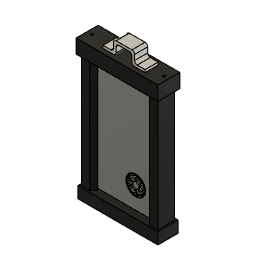
Beskar ingot holder v2 (Autodesk Fusion 360 design; units mm, degrees)
Autodesk Fusion 360 part; units mm, degrees
sketch "Sketch1" plane through (0, 0, 0) normal (0, 1, 0) x (1, 0, 0)
  line L0 (37.5, 3.5) -> (-37.5, 3.5)
  line L1 (-37.5, 3.5) -> (-37.5, -3.5)
  line L2 (-37.5, -3.5) -> (37.5, -3.5)
  line L3 (37.5, -3.5) -> (37.5, 3.5)
  line L4 (37.5, 3.5) -> (-37.5, -3.5) construction
  line L5 (-37.5, 3.5) -> (37.5, -3.5) construction
  line L6 (-43.5, -9.5) -> (43.5, -9.5)
  line L7 (43.5, -9.5) -> (43.5, 9.5)
  line L8 (43.5, 9.5) -> (-43.5, 9.5)
  line L9 (-43.5, 9.5) -> (-43.5, -9.5)
  line L10 (-43.5, 9.5) -> (-36.2124, 9.5)
  line L11 (-36.2124, 9.5) -> (-36.2124, 7.7353)
  line L12 (-36.2124, 7.7353) -> (-43.5, 7.7353)
  line L13 (-43.5, 7.7353) -> (-43.5, 9.5)
  line L14 (-43.5, 9.5) -> (-36.2124, 7.7353) construction
  line L15 (-36.2124, 9.5) -> (-43.5, 7.7353) construction
  line L16 (47, -6) -> (40, -6)
  line L17 (40, -6) -> (40, -13)
  line L18 (40, -13) -> (47, -13)
  line L19 (47, -13) -> (47, -6)
  line L20 (47, -6) -> (40, -13) construction
  line L21 (40, -6) -> (47, -13) construction
  line L22 (47, 6) -> (40, 6)
  line L23 (40, 6) -> (40, 13)
  line L24 (40, 13) -> (47, 13)
  line L25 (47, 13) -> (47, 6)
  line L26 (47, 6) -> (40, 13) construction
  line L27 (40, 6) -> (47, 13) construction
  line L28 (-40, -13) -> (-47, -13)
  line L29 (-47, -13) -> (-47, -6)
  line L30 (-47, -6) -> (-40, -6)
  line L31 (-40, -6) -> (-40, -13)
  line L32 (-40, -13) -> (-47, -6) construction
  line L33 (-47, -13) -> (-40, -6) construction
  line L34 (-40, 6) -> (-47, 6)
  line L35 (-47, 6) -> (-47, 13)
  line L36 (-47, 13) -> (-40, 13)
  line L37 (-40, 13) -> (-40, 6)
  line L38 (-40, 6) -> (-47, 13) construction
  line L39 (-47, 6) -> (-40, 13) construction
  line L40 (0, 0) -> (-0.7931, -0.074)
  circle A0 centre (0, 0) radius 15
  circle A1 centre (15, 0) radius 1.99
  circle A2 centre (-15, 0) radius 1.99
  line L41 (-37.5, 0) -> (-41, 0)
  line L42 (37.5, 0) -> (41, 0)
  circle A3 centre (41, 0) radius 1.5
  circle A4 centre (-41, 0) radius 1.5
  line L43 (-46.5, -12.5) -> (46.5, -12.5)
  line L44 (46.5, -12.5) -> (46.5, 12.5)
  line L45 (46.5, 12.5) -> (-46.5, 12.5)
  line L46 (-46.5, 12.5) -> (-46.5, -12.5)
  point P0 (-39.8562, 8.6177)
  point P1 (43.5, -9.5)
  point P2 (43.5, 9.5)
  point P3 (-43.5, -9.5)
  point P4 (-43.5, 9.5)
  dimension "d1" = 75
  dimension "d2" = 7
  dimension "d3" = 6
  dimension "d4" = 7
  dimension "d5" = 7
  dimension "d6" = 7
  dimension "d7" = 7
  dimension "d8" = 7
  dimension "d9" = 7
  dimension "d10" = 7
  dimension "d11" = 7
  dimension "d26" = 30
  dimension "d27" = 3.98
  dimension "d28" = 3.98
  dimension "d31" = 3.5
  dimension "d32" = 3.5
  dimension "d33" = 3
  dimension "d34" = 3
  dimension "d66" = 9
  constraint horizontal L0
  constraint perpendicular L0 L1
  constraint parallel L0 L2
  constraint parallel L1 L3
  constraint coincident L4 L40.start
  constraint coincident L5 L40.start
  constraint coincident L40.start A0.centre
  constraint horizontal L10
  constraint perpendicular L10 L11
  constraint parallel L10 L12
  constraint parallel L11 L13
  constraint coincident L14 P0
  constraint coincident L15 P0
  constraint horizontal L16
  constraint perpendicular L16 L17
  constraint parallel L16 L18
  constraint parallel L17 L19
  constraint coincident L20 P1
  constraint coincident L21 P1
  constraint coincident P1 L6.end
  constraint horizontal L22
  constraint perpendicular L22 L23
  constraint parallel L22 L24
  constraint parallel L23 L25
  constraint coincident L26 P2
  constraint coincident L27 P2
  constraint coincident P2 L7.end
  constraint horizontal L28
  constraint perpendicular L28 L29
  constraint parallel L28 L30
  constraint parallel L29 L31
  constraint coincident L32 P3
  constraint coincident L33 P3
  constraint coincident P3 L6.start
  constraint horizontal L34
  constraint perpendicular L34 L35
  constraint parallel L34 L36
  constraint parallel L35 L37
  constraint coincident L38 P4
  constraint coincident L39 P4
  constraint coincident P4 L8.end
  constraint coincident L4 L40.end
  constraint coincident A0 A1.centre
  constraint coincident A0 A2.centre
  constraint midpoint L1 L41.start
  constraint perpendicular L1 L41
  constraint midpoint L3 L42.start
  constraint perpendicular L7 L42
  constraint coincident L42.end A3.centre
  constraint coincident L41.end A4.centre
  measures "d1" distance of L1.end L2.end
  measures "d2" distance of L0.end L1.end
  measures "d4" distance of L17.end L18.end
  measures "d5" distance of L16.end L17.end
  measures "d6" distance of L23.end L24.end
  measures "d7" distance of L22.end L23.end
  measures "d8" distance of L29.end L30.end
  measures "d9" distance of L28.end L29.end
  measures "d10" distance of L35.end L36.end
  measures "d11" distance of L34.end L35.end
  measures "d26" diameter of A0
  measures "d27" diameter of A1
  measures "d28" diameter of A2
  measures "d31" distance of L41.start L41.end
  measures "d32" distance of L42.start L42.end
  measures "d33" diameter of A3
  measures "d34" diameter of A4
extrude "Extrude1" add sketch "Sketch1" along normal blind 7 contours L0 L2 L3 L6 L7 L8 L16 L17 L22 L23 A0 | L0 L8 A0 | L0 L1 L2 L6 L8 L9 L11 L12 L30 L31 L34 L37 A0 | L7 L8 L22 L23 | L2 L6 A0 | L8 L10 L11 L12 L37 | L8 L9 L10 L12 L13 L37 | L6 L7 L16 L17 | L9 L12 L34 L37 | L6 L9 L30 L31 | A3 | A4 makes body 1
extrude "Extrude2" add sketch "Sketch1" 1 faces at (-3.8694, 0, 5.5) against normal blind 6 contours L0 L2 L3 A0 A1 | L0 L2 L3 L6 L7 L8 L16 L17 L22 L23 A0 | L0 L2 A0 A1 A2 | L0 L8 A0 | L0 L1 L2 A0 A2 | L0 L1 L2 L6 L8 L9 L11 L12 L30 L31 L34 L37 A0 | A0 A1 | A0 A1 | A0 A2 | A0 A2 | L7 L8 L22 L23 | L2 L6 A0 | L8 L10 L11 L12 L37 | L8 L9 L10 L12 L13 L37 | L6 L7 L16 L17 | L9 L12 L34 L37 | L6 L9 L30 L31 | A3 | A4 on bodies 1 bodies 1
sketch "Sketch2" plane through (0, 7, 0) normal (0, 1, 0) x (-1, 0, 0)
  line L0 (-37.5, -3.5) -> (-37.5, 3.5)
  line L1 (-37.5, 3.5) -> (37.5, 3.5)
  line L2 (37.5, 3.5) -> (37.5, -3.5)
  line L3 (37.5, -3.5) -> (-37.5, -3.5)
  line L4 (43.5, -9.5) -> (43.5, 9.5)
  line L5 (43.5, 9.5) -> (-43.5, 9.5)
  line L6 (-43.5, 9.5) -> (-43.5, -9.5)
  line L7 (-43.5, -9.5) -> (43.5, -9.5)
  line L8 (-43.5, -3.5) -> (43.5, -3.5)
  line L9 (-43.5, 3.5) -> (43.5, 3.5)
  line L10 (-43.5, -5) -> (43.5, -5)
  line L11 (-43.5, 4.9996) -> (43.5, 4.9996)
  line L12 (-37.5, 4.9996) -> (-37.5, -5)
  line L13 (37.5, 4.9996) -> (37.5, -5)
  line L14 (43.5, -9.5) -> (29.5, -9.5)
  line L15 (29.5, -9.5) -> (29.5, 9.5)
  line L16 (29.5, 9.5) -> (43.5, 9.5)
  line L17 (43.5, 9.5) -> (43.5, -9.5)
  line L18 (-43.5, 9.5) -> (-29.5, 9.5)
  line L19 (-29.5, 9.5) -> (-29.5, -9.5)
  line L20 (-29.5, -9.5) -> (-43.5, -9.5)
  line L21 (-43.5, -9.5) -> (-43.5, 9.5)
  dimension "d16" = 1.5
  dimension "d17" = -1.4996
  dimension "d46" = 14
  dimension "d47" = 14
  constraint coincident L6 L8.start
  constraint coincident L4 L8.end
  constraint perpendicular L4 L8
  constraint coincident L6 L9.start
  constraint coincident L4 L9.end
  constraint perpendicular L4 L9
  constraint coincident L11 L12.start
  constraint coincident L10 L12.end
  constraint perpendicular L10 L12
  constraint coincident L11 L13.start
  constraint coincident L10 L13.end
  constraint perpendicular L10 L13
  constraint horizontal L14
  constraint vertical L15
  constraint horizontal L16
  constraint vertical L17
  constraint coincident L4.start L7.end
  constraint horizontal L18
  constraint vertical L19
  constraint horizontal L20
  constraint vertical L21
  constraint coincident L5.end L6.start
  measures "d46" distance of L4.start L14.end
  measures "d47" distance of L5.end L18.end
extrude "Extrude3" add sketch "Sketch2" along normal blind 132.5 separate body contours L0 L6 L8 L9 L12 L21 | L6 L8 L10 L12 L21 | L6 L9 L11 L12 L21 | L6 L7 L10 L19 L20 L21 | L5 L6 L11 L18 L19 L21 | L2 L4 L8 L9 L13 L17 | L4 L8 L10 L13 L17 | L4 L7 L10 L14 L15 L17 | L4 L9 L11 L13 L17 | L4 L5 L11 L15 L16 L17 makes body 2 at (-43.5, 51.1667, -3.1667) makes body 3 at (43.5, 51.1667, 3.1667)
extrude "Extrude4" add sketch "Sketch1" along normal blind 139 separate body contours L0 L2 L3 A0 A1 | L0 L2 A0 A1 A2 | L0 L1 L2 A0 A2 | A0 A1 | A0 A1 | A0 A2 | A0 A2 makes body 4
sketch "Sketch3" plane through (-43.5, 0, 0) normal (-1, 0, 0) x (0, 0, 1)
  line L0 (-9.5, -6) -> (9.5, -6)
  line L1 (-9.5, 142) -> (-4.5002, 142)
  line L2 (-4.5002, 142) -> (-4.5002, 137)
  line L3 (-4.5002, 137) -> (-9.5, 137)
  line L4 (-9.5, 137) -> (-9.5, 142)
  circle A0 centre (-4.5002, 137) radius 1.25
  line L5 (9.5, -6) -> (9.5, 7)
  line L6 (-9.5, 7) -> (-9.5, -6)
  line L7 (9.5, 7) -> (-9.5, 7)
  dimension "d22" = 5
  dimension "d23" = 2.5
  constraint horizontal L1
  constraint vertical L2
  constraint horizontal L3
  constraint vertical L4
  constraint coincident L2.end L3.start
  measures "d22" distance of L1.start L3.end
  measures "d23" diameter of A0
extrude "Extrude5" [suppressed]
extrude "Extrude6" cut sketch "Sketch1" along normal blind 10 and the other way blind 6 contours A3 | A4 bodies 1 3 2
extrude "Extrude7" add sketch "Sketch3" against normal blind 87 separate body contours L2 L3 A0 | L2 L3 A0 makes body 5
sketch "Sketch4" plane through (0, 0, -3.5) normal (0, 0, -1) x (-1, 0, 0)
  line L0 (-37.5, 0) -> (37.5, 0)
  line L1 (37.5, 0) -> (37.5, 139)
  line L2 (37.5, 139) -> (-37.5, 139)
  line L3 (-37.5, 139) -> (-37.5, 0)
  line L4 (-37.5, 139) -> (-12.5, 139)
  line L5 (-12.5, 139) -> (-12.5, 114)
  line L6 (-12.5, 114) -> (-37.5, 114)
  line L7 (-37.5, 114) -> (-37.5, 139)
  spline S0 degree 3 poles (-12.2923, 125.7038) (-6.1064, 125.7038) (-1.086, 120.6834) (-1.086, 114.4975) knots 0 0 0 0 1 1 1 1
  spline S1 degree 3 poles (-1.086, 114.4975) (-1.086, 108.3117) (-6.1064, 103.2912) (-12.2923, 103.2913) knots 0 0 0 0 1 1 1 1
  spline S2 degree 3 poles (-12.2923, 103.2913) (-18.4782, 103.2913) (-23.4986, 108.3117) (-23.4986, 114.4975) knots 0 0 0 0 1 1 1 1
  spline S3 degree 3 poles (-23.4986, 114.4975) (-23.4986, 120.6834) (-18.4782, 125.7038) (-12.2923, 125.7038) knots 0 0 0 0 1 1 1 1
  spline S4 degree 3 poles (-11.7634, 124.7747) (-11.7697, 124.7751) (-11.7762, 124.7744) (-11.7825, 124.7747) knots 0 0 0 0 1 1 1 1
  line L8 (-11.7825, 124.7747) -> (-11.8301, 124.0148)
  spline S5 degree 3 poles (-11.8301, 124.0148) (-11.1838, 123.984) (-10.5547, 123.8897) (-9.9481, 123.7361) knots 0 0 0 0 1 1 1 1
  line L9 (-9.9481, 123.7361) -> (-10.1363, 122.9952)
  spline S6 degree 3 poles (-10.1363, 122.9952) (-8.5442, 122.5919) (-7.1261, 121.7535) (-6.0149, 120.6129) knots 0 0 0 0 1 1 1 1
  line L10 (-6.0149, 120.6129) -> (-5.4694, 121.1465)
  spline S7 degree 3 poles (-5.4694, 121.1465) (-5.0257, 120.6913) (-4.629, 120.1913) (-4.283, 119.6552) knots 0 0 0 0 1 1 1 1
  line L11 (-4.283, 119.6552) -> (-3.6446, 120.0769)
  spline S8 degree 3 poles (-3.6446, 120.0769) (-5.3883, 122.773) (-8.3585, 124.602) (-11.7634, 124.7747) knots 0 0 0 0 1 1 1 1
  spline S9 degree 3 poles (-12.8021, 124.7747) (-16.2149, 124.6078) (-19.193, 122.778) (-20.94, 120.0769) knots 0 0 0 0 1 1 1 1
  line L12 (-20.94, 120.0769) -> (-20.3015, 119.6552)
  spline S10 degree 3 poles (-20.3015, 119.6552) (-19.9563, 120.19) (-19.56, 120.6899) (-19.1175, 121.1441) knots 0 0 0 0 1 1 1 1
  line L13 (-19.1175, 121.1441) -> (-18.572, 120.6129)
  spline S11 degree 3 poles (-18.572, 120.6129) (-17.4607, 121.7541) (-16.0409, 122.5918) (-14.4483, 122.9952) knots 0 0 0 0 1 1 1 1
  line L14 (-14.4483, 122.9952) -> (-14.6365, 123.7361)
  spline S12 degree 3 poles (-14.6365, 123.7361) (-14.0299, 123.8897) (-13.4008, 123.984) (-12.7544, 124.0148) knots 0 0 0 0 1 1 1 1
  line L15 (-12.7544, 124.0148) -> (-12.8021, 124.7747)
  spline S13 degree 3 poles (-12.2923, 121.4157) (-12.6163, 121.4165) (-12.9403, 121.3967) (-13.2071, 121.3585) knots 0 0 0 0 1 1 1 1
  line L16 (-13.2071, 121.3585) -> (-12.7902, 117.8899)
  spline S14 degree 3 poles (-12.7902, 117.8899) (-13.6665, 117.7621) (-14.4348, 117.3035) (-14.9652, 116.644) knots 0 0 0 0 1 1 1 1
  line L17 (-14.9652, 116.644) -> (-17.7477, 118.7309)
  spline S15 degree 3 poles (-17.7477, 118.7309) (-18.0857, 118.3098) (-18.4689, 117.6493) (-18.6697, 117.149) knots 0 0 0 0 1 1 1 1
  line L18 (-18.6697, 117.149) -> (-15.4726, 115.7816)
  spline S16 degree 3 poles (-15.4726, 115.7816) (-15.6333, 115.3846) (-15.7228, 114.952) (-15.7228, 114.4975) knots 0 0 0 0 1 1 1 1
  spline S17 degree 3 poles (-15.7228, 114.4975) (-15.7228, 114.0598) (-15.6414, 113.6414) (-15.4917, 113.2564) knots 0 0 0 0 1 1 1 1
  line L19 (-15.4917, 113.2564) -> (-18.6625, 111.9008)
  spline S18 degree 3 poles (-18.6625, 111.9008) (-18.4669, 111.3976) (-18.0877, 110.7383) (-17.7549, 110.3142) knots 0 0 0 0 1 1 1 1
  line L20 (-17.7549, 110.3142) -> (-14.9914, 112.3821)
  spline S19 degree 3 poles (-14.9914, 112.3821) (-14.4617, 111.7075) (-13.6846, 111.2364) (-12.7973, 111.1052) knots 0 0 0 0 1 1 1 1
  line L21 (-12.7973, 111.1052) -> (-13.2071, 107.6937)
  spline S20 degree 3 poles (-13.2071, 107.6937) (-12.6735, 107.6115) (-11.9111, 107.6127) (-11.3775, 107.689) knots 0 0 0 0 1 1 1 1
  line L22 (-11.3775, 107.689) -> (-11.7872, 111.1052)
  spline S21 degree 3 poles (-11.7872, 111.1052) (-10.8993, 111.2365) (-10.1229, 111.7091) (-9.5931, 112.3845) knots 0 0 0 0 1 1 1 1
  line L23 (-9.5931, 112.3845) -> (-6.8368, 110.3166)
  spline S22 degree 3 poles (-6.8368, 110.3166) (-6.4989, 110.7377) (-6.1157, 111.3982) (-5.9149, 111.8985) knots 0 0 0 0 1 1 1 1
  line L24 (-5.9149, 111.8985) -> (-9.0929, 113.2588)
  spline S23 degree 3 poles (-9.0929, 113.2588) (-8.9437, 113.6432) (-8.8618, 114.0606) (-8.8618, 114.4975) knots 0 0 0 0 1 1 1 1
  spline S24 degree 3 poles (-8.8618, 114.4975) (-8.8618, 114.9527) (-8.9507, 115.3864) (-9.1119, 115.784) knots 0 0 0 0 1 1 1 1
  line L25 (-9.1119, 115.784) -> (-5.922, 117.1467)
  spline S25 degree 3 poles (-5.922, 117.1467) (-6.1177, 117.6499) (-6.4969, 118.3092) (-6.8297, 118.7333) knots 0 0 0 0 1 1 1 1
  line L26 (-6.8297, 118.7333) -> (-9.6194, 116.644)
  spline S26 degree 3 poles (-9.6194, 116.644) (-10.1498, 117.3035) (-10.9181, 117.7621) (-11.7944, 117.8899) knots 0 0 0 0 1 1 1 1
  line L27 (-11.7944, 117.8899) -> (-11.3775, 121.3538)
  spline S27 degree 3 poles (-11.3775, 121.3538) (-11.6443, 121.3949) (-11.9683, 121.415) (-12.2923, 121.4157) knots 0 0 0 0 1 1 1 1
  line L28 (-3.1348, 119.1954) -> (-3.8209, 118.8571)
  spline S28 degree 3 poles (-3.8209, 118.8571) (-3.5315, 118.2961) (-3.2949, 117.7038) (-3.1205, 117.0847) knots 0 0 0 0 1 1 1 1
  line L29 (-3.1205, 117.0847) -> (-3.8542, 116.8775)
  spline S29 degree 3 poles (-3.8542, 116.8775) (-3.6409, 116.1205) (-3.5255, 115.3225) (-3.5255, 114.4975) knots 0 0 0 0 1 1 1 1
  spline S30 degree 3 poles (-3.5255, 114.4975) (-3.5255, 113.6718) (-3.6405, 112.8729) (-3.8542, 112.1153) knots 0 0 0 0 1 1 1 1
  line L30 (-3.8542, 112.1153) -> (-3.1205, 111.908)
  spline S31 degree 3 poles (-3.1205, 111.908) (-3.2948, 111.2899) (-3.5318, 110.6981) (-3.8209, 110.138) knots 0 0 0 0 1 1 1 1
  line L31 (-3.8209, 110.138) -> (-3.1348, 109.7997)
  spline S32 degree 3 poles (-3.1348, 109.7997) (-2.4102, 111.2083) (-2.0008, 112.8054) (-2.0008, 114.4975) knots 0 0 0 0 1 1 1 1
  spline S33 degree 3 poles (-2.0008, 114.4975) (-2.0008, 116.1897) (-2.4102, 117.7867) (-3.1348, 119.1954) knots 0 0 0 0 1 1 1 1
  spline S34 degree 3 poles (-21.4498, 119.1954) (-22.1744, 117.7867) (-22.5838, 116.1897) (-22.5838, 114.4975) knots 0 0 0 0 1 1 1 1
  spline S35 degree 3 poles (-22.5838, 114.4975) (-22.5838, 112.8054) (-22.1744, 111.2083) (-21.4498, 109.7997) knots 0 0 0 0 1 1 1 1
  line L32 (-21.4498, 109.7997) -> (-20.7637, 110.138)
  spline S36 degree 3 poles (-20.7637, 110.138) (-21.0529, 110.6983) (-21.2897, 111.2897) (-21.4641, 111.908) knots 0 0 0 0 1 1 1 1
  line L33 (-21.4641, 111.908) -> (-20.7304, 112.1153)
  spline S37 degree 3 poles (-20.7304, 112.1153) (-20.9441, 112.8729) (-21.0591, 113.6718) (-21.0591, 114.4975) knots 0 0 0 0 1 1 1 1
  spline S38 degree 3 poles (-21.0591, 114.4975) (-21.0591, 115.3225) (-20.9437, 116.1205) (-20.7304, 116.8775) knots 0 0 0 0 1 1 1 1
  line L34 (-20.7304, 116.8775) -> (-21.4641, 117.0847)
  spline S39 degree 3 poles (-21.4641, 117.0847) (-21.2897, 117.7037) (-21.053, 118.2963) (-20.7637, 118.8571) knots 0 0 0 0 1 1 1 1
  line L35 (-20.7637, 118.8571) -> (-21.4498, 119.1954)
  spline S40 degree 3 poles (-4.283, 109.3399) (-4.6291, 108.8038) (-5.0257, 108.3038) (-5.4694, 107.8486) knots 0 0 0 0 1 1 1 1
  line L36 (-5.4694, 107.8486) -> (-6.0149, 108.3822)
  spline S41 degree 3 poles (-6.0149, 108.3822) (-7.1261, 107.2416) (-8.5442, 106.4032) (-10.1363, 105.9999) knots 0 0 0 0 1 1 1 1
  line L37 (-10.1363, 105.9999) -> (-9.9481, 105.259)
  spline S42 degree 3 poles (-9.9481, 105.259) (-10.5547, 105.1054) (-11.1838, 105.0111) (-11.8301, 104.9803) knots 0 0 0 0 1 1 1 1
  line L38 (-11.8301, 104.9803) -> (-11.7825, 104.2203)
  spline S43 degree 3 poles (-11.7825, 104.2203) (-8.3697, 104.3873) (-5.3915, 106.2171) (-3.6446, 108.9182) knots 0 0 0 0 1 1 1 1
  line L39 (-3.6446, 108.9182) -> (-4.283, 109.3399)
  line L40 (-20.3039, 109.3399) -> (-20.94, 108.9182)
  spline S44 degree 3 poles (-20.94, 108.9182) (-19.193, 106.2171) (-16.2149, 104.3873) (-12.8021, 104.2203) knots 0 0 0 0 1 1 1 1
  line L41 (-12.8021, 104.2203) -> (-12.7544, 104.9803)
  spline S45 degree 3 poles (-12.7544, 104.9803) (-13.4008, 105.0111) (-14.0299, 105.1054) (-14.6365, 105.259) knots 0 0 0 0 1 1 1 1
  line L42 (-14.6365, 105.259) -> (-14.4483, 105.9999)
  spline S46 degree 3 poles (-14.4483, 105.9999) (-16.0409, 106.4033) (-17.4607, 107.241) (-18.572, 108.3822) knots 0 0 0 0 1 1 1 1
  line L43 (-18.572, 108.3822) -> (-19.1175, 107.851)
  spline S47 degree 3 poles (-19.1175, 107.851) (-19.5606, 108.3058) (-19.9583, 108.8044) (-20.3039, 109.3399) knots 0 0 0 0 1 1 1 1
  dimension "d71" = 25
  dimension "d72" = 25
  constraint horizontal L4
  constraint vertical L5
  constraint horizontal L6
  constraint vertical L7
  constraint coincident L2.end L3.start
  measures "d71" distance of L2.end L4.end
  measures "d72" distance of L2.end L6.end
extrude "Extrude8" cut sketch "Sketch4" against normal blind 2 contours L5 L6 S2 S3 S13 L16 S14 L17 S15 L18 S16 S17 S34 S35 S37 S38 L34 S39 L35 | L5 L6 S0 S1 S2 S3 S13 S17 L19 S18 L20 S19 L21 S20 L22 S21 L23 S22 L24 S23 S24 L25 S25 L26 S26 L27 S27 S35 L32 S36 L33 S37 bodies 4
sketch "Sketch5" plane through (0, 7, 0) normal (0, 1, 0) x (-1, 0, 0)
sketch "Sketch6" plane through (0, 0, -3.5) normal (0, 0, -1) x (1, 0, 0)
  line L0 (-41.075, 0) -> (-41.075, -10)
  line L1 (-41.075, -10) -> (40.7156, -10)
  line L2 (40.7156, -10) -> (40.7156, 0)
  line L3 (40.7156, 0) -> (37.052, 1.1708)
  dimension "d39" = 10
  constraint perpendicular L0 L1
  measures "d39" distance of L0.start L0.end
pipe "Pipe1" add diameter 2 path "Sketch6" along L0 L1 L2 L3 separate body makes body 6
move_body "Move1" bodies 6 to x (1, 0, 0) y (0, 1, 0) z (0, 0, 1) at (0, -15, 0)
move_body "Move2" bodies 6 to x (-1, 0, 0) y (0, -1, 0) z (0, 0, 1) at (-0.1499, -19.2466, 4)
chamfer "Chamfer1" distance 4.5 angle 45 2 edges at (-29.5, 73.25, -9.5) (29.5, 73.25, -9.5) on bodies 2 3
chamfer "Chamfer1" distance 4.5 angle 45 2 edges at (29.5, 73.25, 9.5) (-29.5, 73.25, 9.5) on bodies 2 3
sketch "Sketch7" plane through (-43.5, 0, 0) normal (-1, 0, 0) x (0, 0, 1)
  line L0 (-9.5, 7) -> (-9.5, -6)
  line L1 (-9.5, -6) -> (9.5, -6)
  line L2 (9.5, -6) -> (9.5, 7)
  line L3 (9.5, 7) -> (-9.5, 7)
sketch "Sketch8" plane through (0, 139.5, 0) normal (0, 1, 0) x (-1, 0, 0)
  line L0 (34, 9.5) -> (29.5, 5)
  line L1 (29.5, 5) -> (29.5, 4.9996)
  line L2 (29.5, 4.9996) -> (37.5, 4.9996)
  line L3 (37.5, 4.9996) -> (37.5, -5)
  line L4 (37.5, -5) -> (29.5, -5)
  line L5 (29.5, -5) -> (34, -9.5)
  line L6 (34, -9.5) -> (43.5, -9.5)
  line L7 (43.5, -9.5) -> (43.5, 9.5)
  line L8 (43.5, 9.5) -> (34, 9.5)
  line L9 (43.5, -9.5) -> (-43.5, -9.5)
  line L10 (-43.5, -9.5) -> (-43.5, 9.5)
  line L11 (-43.5, 9.5) -> (43.5, 9.5)
  line L12 (43.5, 9.5) -> (43.5, -9.5)
  line L13 (-45.5, 11.5) -> (45.5, 11.5)
  line L14 (45.5, 11.5) -> (45.5, -11.5)
  line L15 (45.5, -11.5) -> (-45.5, -11.5)
  line L16 (-45.5, -11.5) -> (-45.5, 11.5)
  line L17 (43.5, 0) -> (40.5, 0)
  line L18 (-43.5, 0) -> (-40.5, 0)
  circle A0 centre (-40.5, 0) radius 1.52
  circle A1 centre (40.5, 0) radius 1.52
  line L19 (40.5, 0) -> (40.5, 5)
  circle A2 centre (40.5, 5) radius 1.375
  line L20 (-40.5, 0) -> (-40.5, 5)
  circle A3 centre (-40.5, 5) radius 1.375
  point P0 (-41, -2)
  dimension "d50" = -2
  dimension "d53" = 3
  dimension "d54" = 3
  dimension "d55" = 3.04
  dimension "d56" = 3.04
  dimension "d99" = 5
  dimension "d100" = 2.75
  dimension "d103" = 5
  dimension "d104" = 2.75
  constraint horizontal L9
  constraint vertical L10
  constraint horizontal L11
  constraint vertical L12
  constraint coincident L6.end L7.start
  constraint horizontal L17
  constraint midpoint L12 L17.start
  constraint midpoint L10 L18.start
  constraint perpendicular L10 L18
  constraint coincident L18.end A0.centre
  constraint coincident L17.end A1.centre
  constraint parallel L14 L19
  constraint coincident L19.end A2.centre
  constraint perpendicular L18 L20
  constraint coincident L20.end A3.centre
  measures "d53" distance of L17.start L17.end
  measures "d54" distance of L18.start L18.end
  measures "d55" diameter of A0
  measures "d56" diameter of A1
  measures "d99" distance of L17.end L19.end
  measures "d100" diameter of A2
  measures "d103" distance of L18.end L20.end
  measures "d104" diameter of A3
extrude "Extrude9" add sketch "Sketch8" along normal blind 13 separate body contours L0 L2 L3 L4 L5 L6 L7 L8 L9 L11 L12 | L0 L2 L3 L4 L5 L9 L10 L11 | L13 L14 L15 L16 | L17 A1 L19 | L17 A1 L19 | L18 A0 L20 | L18 A0 L20 | A2 | A3 makes body 7
extrude "Extrude10" cut sketch "Sketch8" along normal blind 16 and the other way blind 3 contours L17 A1 L19 | L17 A1 L19 | L18 A0 L20 | L18 A0 L20 bodies 7 1 3 2
extrude "Extrude11" cut sketch "Sketch1" along normal blind 5.7 from surface at -6 contours A0 A1 | A0 A1 | A0 A2 | A0 A2 bodies 1
extrude "Extrude12" add sketch "Sketch1" along normal blind 10 and the other way blind 6 contours L8 L23 A0 L45 | L8 A0 L45 | L8 L10 L37 A0 L45 | L7 L8 L22 L23 L44 L45 | L6 A0 L43 | L6 L17 A0 L43 | L8 L9 L10 L13 L34 L37 L45 L46 | L7 L16 L22 L44 | L6 L31 A0 L43 | L6 L7 L16 L17 L43 L44 | L6 L9 L30 L31 L43 L46 | L9 L30 L34 L46 bodies 1
sketch "Sketch9" plane through (0, 0, 0) normal (0, 0, 1) x (1, 0, 0)
  line L0 (-15.0557, -6, -12.5) -> (14.9443, -6, -12.5)
  line L1 (14.9443, -12, -12.5) -> (14.9443, -21, -12.5)
  line L2 (14.9443, -21, -12.5) -> (-15.0557, -21, -12.5)
  line L3 (-15.0557, -21, -12.5) -> (-15.0557, -6, -12.5)
  line L4 (-46.5, -6, -12.5) -> (46.5, -6, -12.5)
  line L5 (-15.0557, -21, -12.5) -> (-9.0557, -21, -12.5)
  line L6 (-9.0557, -21, -12.5) -> (-9.0557, -6, -12.5)
  line L7 (-9.0557, -6, -12.5) -> (-15.0557, -6, -12.5)
  line L8 (-15.0557, -6, -12.5) -> (-15.0557, -21, -12.5)
  line L9 (14.9443, -21, -12.5) -> (20.9443, -21, -12.5)
  line L10 (20.9443, -21, -12.5) -> (20.9443, -6, -12.5)
  line L11 (20.9443, -6, -12.5) -> (14.9443, -6, -12.5)
  line L12 (14.9443, -6, -12.5) -> (14.9443, -21, -12.5)
  line L13 (-9.0557, -6, -12.5) -> (-21.0557, -6, -12.5)
  line L14 (-21.0557, -6, -12.5) -> (-21.0557, -9, -12.5)
  line L15 (-21.0557, -9, -12.5) -> (-12.0557, -9, -12.5)
  line L16 (-9.0557, -9, -12.5) -> (-9.0557, -6, -12.5)
  line L17 (15, -6) -> (27, -6)
  line L18 (27, -6) -> (27, -9)
  line L19 (27, -9) -> (15, -9)
  line L20 (15, -9) -> (15, -6)
  line L21 (-9.0557, -6, -12.5) -> (905.3443, -6, -12.5)
  line L22 (905.3443, -6, -12.5) -> (905.3443, -21, -12.5)
  line L23 (905.3443, -21, -12.5) -> (-9.0557, -21, -12.5)
  line L24 (-9.0557, -18, -12.5) -> (-9.0557, -12, -12.5)
  line L25 (-9.0557, -6, -12.5) -> (-9.0557, -6, -12.5)
  line L26 (-6.0557, -9, -12.5) -> (-6.0557, -15, -12.5)
  line L27 (-6.0557, -21, -12.5) -> (-6.0557, -21, -12.5)
  line L28 (-9.0557, -21, -12.5) -> (-9.0557, -6, -12.5)
  line L29 (14.9443, -6, -12.5) -> (14.9443, -6, -12.5)
  line L30 (11.9443, -9, -12.5) -> (11.9443, -15, -12.5)
  line L31 (11.9443, -21, -12.5) -> (14.9443, -21, -12.5)
  line L32 (14.9443, -21, -12.5) -> (14.9443, -6, -12.5)
  line L33 (-9.0557, -21, -12.5) -> (11.9443, -21, -12.5)
  line L34 (14.9443, -18, -12.5) -> (14.9443, -18, -12.5)
  line L35 (8.9443, -18, -12.5) -> (-3.0557, -18, -12.5)
  line L36 (-9.0557, -18, -12.5) -> (-9.0557, -21, -12.5)
  arc A0 through (-6.0557, -9, -12.5) (-6.9344, -6.8787, -12.5) (-9.0557, -6, -12.5)
  arc A1 through (14.9443, -6, -12.5) (12.823, -6.8787, -12.5) (11.9443, -9, -12.5)
  arc A2 through (11.9443, -21, -12.5) (14.0656, -20.1213, -12.5) (14.9443, -18, -12.5)
  arc A3 through (-9.0557, -18, -12.5) (-8.177, -20.1213, -12.5) (-6.0557, -21, -12.5)
  arc A4 through (-6.0557, -15, -12.5) (-5.177, -17.1213, -12.5) (-3.0557, -18, -12.5)
  arc A5 through (8.9443, -18, -12.5) (11.0656, -17.1213, -12.5) (11.9443, -15, -12.5)
  line L37 (17.9443, -9, -12.5) -> (26.9443, -9, -12.5)
  line L38 (26.9443, -9, -12.5) -> (26.9443, -6, -12.5)
  line L39 (26.9443, -6, -12.5) -> (14.9443, -6, -12.5)
  line L40 (14.9443, -6, -12.5) -> (14.9443, -9, -12.5)
  arc A6 through (17.9443, -9, -12.5) (15.823, -9.8787, -12.5) (14.9443, -12, -12.5)
  arc A7 through (-9.0557, -12, -12.5) (-9.9344, -9.8787, -12.5) (-12.0557, -9, -12.5)
  point P0 (-6.0557, -6)
  point P1 (11.9443, -6)
  dimension "d73" = 30
  dimension "d74" = 15
  dimension "d75" = 6
  dimension "d76" = 15
  dimension "d77" = 6
  dimension "d78" = 15
  dimension "d79" = 12
  dimension "d80" = 3
  dimension "d81" = 12
  dimension "d82" = 3
  dimension "d83" = 914.4
  dimension "d84" = 3
  dimension "d85" = 3
  dimension "d86" = 3
  dimension "d87" = 3
  dimension "d88" = 3
  dimension "d89" = 3
  dimension "d90" = 3
  dimension "d91" = 3
  dimension "d92" = 3
  dimension "d93" = 12
  dimension "d94" = 3
  dimension "d95" = 3
  constraint horizontal L17
  constraint vertical L18
  constraint horizontal L19
  constraint vertical L20
  measures "d81" distance of L17.start L17.end
  measures "d82" distance of L17.start L19.end
extrude "Extrude13" add sketch "Sketch9" along normal blind 15 from surface at 5 separate body contours L0 L3 L4 L6 L7 L8 L13 L15 L16 L28 A7 | L3 L4 L8 L13 L14 L15 | L1 L2 L6 L12 L16 L23 L24 L26 L28 L30 L32 L33 L35 A0 A1 A2 A3 A4 A5 L40 | L4 L10 L11 L12 L21 L32 L37 L39 L40 A6 | L4 L10 L21 L37 L38 L39 in plane through (0, 0, -12.5) normal (0, 0, 1) makes body 8
extrude "Extrude14" cut sketch "Sketch8" along normal blind 10 and the other way blind 135 contours A2 | A3 bodies 1 2 3 7
move_body "Move3" bodies 1 3 7 2 4 8 to x (1, 0, 0) y (0, -1, 0) z (0, 0, -1) at (0, 20, 0)
hidden bodies 5 6
equation "d66 = 6 mm + 3 mm"
equation "d83 = 3'-0\""
named bodies: "top", "ingot", "LEFT RAIL", "RIGHT RAIL", "bottom"
